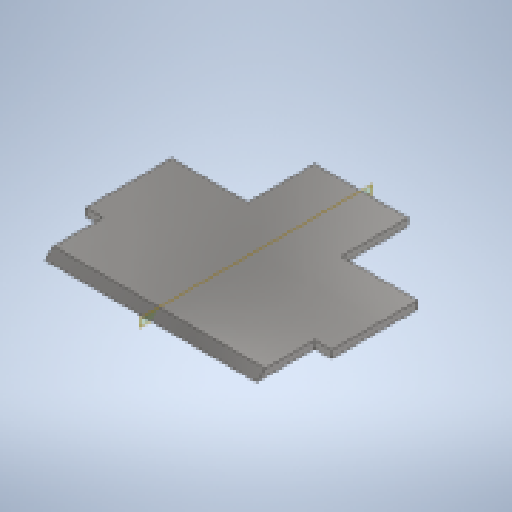
# Autodesk Inventor part: podstawa
Saved by Autodesk Inventor 2023 (Build 270158000, 158)
## iProperties
Created: 2025-01-11
Part Number: podstawa
Material: Stal, odlew
Document SubType Name: Modeling
Designer: kamil
Density: 7.85 g/cm^3
Appearance: Częściowo polerowany
Mass: 153.777 g
Surface Area: 143.041 cm^2
Volume: 19.5894 cm^3
Author: kamil
Autodesk Inventor part; units mm, degrees
ref_plane "YZ Plane" through (0, 0, 0) normal (1, 0, 0) x (0, 1, 0)
ref_plane "XZ Plane" through (0, 0, 0) normal (0, 1, 0) x (-1, 0, 0)
ref_plane "XY Plane" through (0, 0, 0) normal (0, 0, 1) x (1, 0, 0)
sketch "Szkic1" plane through (0, 0, 0) normal (0, 1, 0) x (-1, 0, 0)
  line L0 (50, 50) -> (-50, 50)
  line L1 (-50, 50) -> (-50, -50)
  line L2 (-50, -50) -> (50, -50)
  line L3 (50, -50) -> (50, 50)
  line L4 (50, 50) -> (-50, -50) construction
  line L5 (-50, 50) -> (50, -50) construction
  point P0 (0, 0)
  dimension "d0" = 100
  dimension "d1" = 100
  constraints: 12 end point, 2 midpoint, 2 parallel, 1 horizontal, 1 perpendicular
  measures "d0" distance of L2.end L1.end
  measures "d1" distance of L1.end L0.end
extrude "Wyciągnięcie proste1" add sketch "Szkic1" along normal blind 3
sketch "Szkic2" plane through (0, 3, 0) normal (0, 1, 0) x (1, 0, 0)
  line L0 (50, -50) -> (50, 50) projected
  line L1 (50, 50) -> (-50, 50) projected
  line L2 (-50, 50) -> (-50, -50) projected
  line L3 (-50, -50) -> (50, -50) projected
  line L4 (-50, 50) -> (-19, 50)
  line L5 (-19, 50) -> (-19, 17)
  line L6 (-19, 17) -> (-50, 17)
  line L7 (-50, 17) -> (-50, 50)
  line L8 (50, 50) -> (19, 50)
  line L9 (19, 50) -> (19, 17)
  line L10 (19, 17) -> (50, 17)
  line L11 (50, 17) -> (50, 50)
  point P0 (0, 0)
  dimension "d4" = 31
  dimension "d5" = 33
  dimension "d6" = 31
  constraints: 16 end point, 4 parallel, 2 horizontal, 2 perpendicular, 1 horizontal alignment
  measures "d4" distance of L5.end L6.end
  measures "d5" distance of L4.end L5.end
  measures "d6" distance of L10.end L9.end
extrude "Wyciągnięcie proste2" cut sketch "Szkic2" against normal through all contours L10 L9 L1 L0 | L2 L1 L5 L6
sketch "Szkic3" plane through (0, 3, 0) normal (0, 1, 0) x (1, 0, 0)
  line L0 (19, 17) -> (19, 50) projected
  line L1 (19, 50) -> (-19, 50) projected
  line L2 (-19, 50) -> (-19, 17) projected
  line L3 (-19, 17) -> (-50, 17) projected
  line L4 (-50, 17) -> (-50, -50) projected
  line L5 (-50, -50) -> (50, -50) projected
  line L6 (50, -50) -> (50, 17) projected
  line L7 (50, 17) -> (19, 17) projected
  line L8 (19, 50) -> (-19, 50)
  line L9 (-19, 50) -> (-19, 44)
  line L10 (-19, 44) -> (19, 44)
  line L11 (19, 44) -> (19, 50)
  point P0 (0, 0)
  dimension "d9" = 6
  constraints: 8 end point, 2 parallel, 1 horizontal, 1 perpendicular, 1 point on line
  measures "d9" distance of L9.end L8.end
extrude "Wyciągnięcie proste3" cut sketch "Szkic3" against normal through all contours L10 L2 L1 L0
fillet "Zaokrąglenie1" radius 2 1 edges at (0, 0, -44)
sketch "Szkic5" plane through (-50, 0, 50) normal (-1, 0, 0) x (0, 0, 1)
  line L0 (0, 0) -> (0, 3) projected
  line L1 (-67, 3) -> (-67, 0) projected
  line L2 (-67, 0) -> (0, 0) projected
  line L3 (0, 0) -> (0, 3) projected
  line L4 (-67, 3) -> (0, 3) projected
  line L5 (-4.6672, -3.25) -> (-21.0795, 10.5216) projected
  point P0 (-50, 0)
  point P1 (-12.1156, 3)
  point P2 (-8.5404, 0)
extrude "Wyciągnięcie proste5" cut sketch "Szkic5" against normal through all contours L2 L5 L4 L0
sketch "Szkic6" plane through (0, 0, 0) normal (0, -1, 0) x (1, 0, 0)
  line L0 (-50, 17.8844) -> (-43, 17.8844) projected
  line L1 (-50, 17.8844) -> (-43, 17.8844)
  line L2 (-43, 17.8844) -> (-43, 43.0531)
  line L3 (-43, 43.0531) -> (-50, 43.0531)
  line L4 (-50, 43.0531) -> (-50, 17.8844)
  point P0 (0, 0)
  constraints: 8 end point, 2 parallel, 1 horizontal, 1 perpendicular
extrude "Wyciągnięcie proste6" cut sketch "Szkic6" against normal through all
ref_plane "Płaszczyzna konstrukcyjna1" through (0, 0, -17) normal (-1, 0, 0) x (0, 0, 1)
mirror "Odbij1" about plane through (0, 0, -17) normal (-1, 0, 0) of "Wyciągnięcie proste6"
